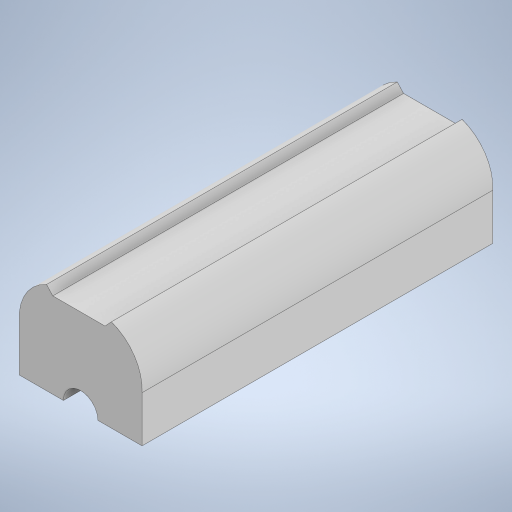
# Autodesk Inventor part: arm rest final 1
Saved by Autodesk Inventor 2023 (Build 270158000, 158)
## iProperties
Created: 2023-10-25
Part Number: arm rest final 1
Material: Generic
Document SubType Name: Modeling
Designer: rachi
Density: 1 g/cm^3
Appearance: Default
Author: rachi
Autodesk Inventor part; units mm, degrees
ref_plane "YZ Plane" through (0, 0, 0) normal (1, 0, 0) x (0, 1, 0)
ref_plane "XZ Plane" through (0, 0, 0) normal (0, 1, 0) x (-1, 0, 0)
ref_plane "XY Plane" through (0, 0, 0) normal (0, 0, 1) x (1, 0, 0)
sketch "Sketch1" plane through (0, 0, 0) normal (0, 0, 1) x (1, 0, 0)
  line L0 (0, 0) -> (40, 0)
  line L1 (40, 0) -> (40, 30)
  line L2 (0, 0) -> (-40, 0)
  line L3 (-40, 0) -> (-40, 30)
  arc A0 (-22.225, 60) -> (-40, 30) centre (-10.109, 32.5554) ccw
  arc A1 (40, 30) -> (20, 60) centre (10.0481, 31.6988) ccw
  line L4 (-22.225, 60) -> (-18.1866, 55.5625)
  line L5 (20, 60) -> (15.875, 55.5625)
  line L6 (-18.1866, 55.5625) -> (15.875, 55.5625)
  circle A2 centre (0, 0) radius 11.25
  point P0 (0, 20)
  point P1 (-11.25, 0)
  point P2 (11.25, 0)
  dimension "d0" = 40
  dimension "d1" = 30
  dimension "d2" = 40
  dimension "d3" = 30
  dimension "d4" = 30
  dimension "d5" = 60
  dimension "d7" = 6
  dimension "d9" = 20
  dimension "d10" = 22.5
  constraints: 14 end point, 4 point on circle, 3 centre point, 3 horizontal, 1 coincident, 1 perpendicular, 1 vertical
  measures "d0" distance of L0.start L0.end
  measures "d1" distance of L0.end L1.end
  measures "d2" distance of L0.start L2.end
  measures "d3" radius of A0
  measures "d4" radius of A1
  measures "d5" distance from line of L2 L4.start
  measures "d7" distance of L4.start L4.end
  measures "d9" distance of point (0, 20) L0.start
  measures "d10" diameter of A2
extrude "Extrusion1" add sketch "Sketch1" along normal blind 228.6 contours A2 L2 L3 A0 L4 L6 L5 A1 L1 L0
body "Solid1"
